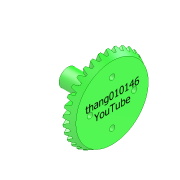
# Autodesk Inventor part: Bevel32x2i2
Saved by Autodesk Inventor 2022.5 (Build 265521000, 521)
## iProperties
Created: 2011-06-16
Part Number: Bevel32x2i2
Document SubType Name: Modeling
Designer: nguyenducthang
Density: 1 g/cm^3
Mass: 34.1157 g
Surface Area: 133.346 cm^2
Volume: 34.1157 cm^3
Material: Generic
Appearance: LED - Green On
Author: nguyenducthang
Autodesk Inventor part; units mm, degrees
ref_plane "YZ Plane" through (0, 0, 0) normal (1, 0, 0) x (0, 1, 0)
sketch "Sketch1" plane through (0, 0, 0) normal (0, 0, 1) x (1, 0, 0)
  line L0 (0, 0) -> (18.861541, 37.723166) construction
  circle A0 centre (0, 0) radius 40 construction
  line L1 (24, 32.721366) -> (16.099657, 36.671529)
  line L2 (21.641182, 47.754605) -> (4.383231, 13.238626) construction
  line L3 (12.405483, 19.444448) -> (19.776293, 34.186101) construction
  line L4 (18, 24.541025) -> (12.073062, 27.504487)
  line L5 (16.099657, 36.671529) -> (16.077282, 36.62678)
  line L6 (0, 0) -> (32.983598, 0) construction
  line L7 (40, 0) -> (43.641618, 0) construction
  line L8 (32.983598, 0) -> (54.544317, 0)
  line L9 (16.077282, 36.62678) -> (12.073062, 27.504487)
  line L10 (18, 24.541025) -> (18, 0)
  line L11 (24, 32.721366) -> (24, 0)
  line L12 (12.073062, 27.504487) -> (0, 0) construction
  line L13 (17.888512, 35.777104) -> (33.472121, 35.777104) construction
  line L14 (17.888512, 35.777104) -> (17.888512, -0.758366) construction
  line L15 (18, 0) -> (24, 0)
  dimension "d0" = 80
  dimension "d2" = 2
  dimension "d3" = 2.4
  dimension "d5" = 10
  dimension "d9" = 40
  dimension "d74" = 63.435
  dimension "d75" = 18
  dimension "d76" = 24
  dimension "d77" = 35.7771
  dimension "d78" = 17.88851
  dimension "d109" = 6.11149
  constraints: 32 end point, 7 perpendicular, 4 collinear, 4 point on line, 3 point on circle, 2 horizontal, 1 centre point, 1 coincident, 1 parallel, 1 tangent, 1 other
  measures "d0" diameter of A0
  measures "d2" distance between parallel lines of L2 L0
  measures "d3" distance between parallel lines of L3 L0
  measures "d5" distance between parallel lines of L4 L1
  measures "d9" distance from line of L1 A0.centre
  measures "d74" angle of L6 L0
  measures "d75" distance from line of L10 A0.centre
  measures "d76" distance from line of L11 A0.centre
  measures "d77" distance between parallel lines of L13 L6
  measures "d78" distance from line of L0.start L14
  measures "d109" distance between parallel lines of L11 L14
sketch "Sketch1 outline for Revolution1" plane through (0, 0, 0) normal (0, 0, 1) x (1, 0, 0)
  line L0 (16.099657, 36.671529) -> (24, 32.721366)
  line L1 (24, 32.721366) -> (24, 0)
  line L2 (24, 0) -> (18, 0)
  line L3 (18, 0) -> (18, 24.541025)
  line L4 (18, 24.541025) -> (12.073062, 27.504487)
  line L5 (12.073062, 27.504487) -> (16.077282, 36.62678)
  line L6 (16.077282, 36.62678) -> (16.099657, 36.671529)
revolve "Revolution1" add sketch "Sketch1 outline for Revolution1" angle 360 about axis through (32.983598, 0, 0) along (1, 0, 0)
ref_plane "Work Plane7" through (17.888512, 35.777104, 0) normal (0.4472128, 0.8944276, 0) x (0, 0, 1)
ref_plane "Work Plane6" through (0, 0, 0) normal (0.4472128, 0.8944276, 0) x (0, 0, 1)
sketch "Sketch11" plane through (17.888512, 35.777104, 0) normal (0.4472128, 0.8944276, 0) x (0, 0, 1)
  ellipse E0 centre (0, 14.399977) end of major axis (36.671529, 14.399977) minor radius 16.399977
  line L0 (0, 14.399977) -> (0, -5.22706) construction
  line L1 (0, -2) -> (-19.262991, -2) construction
  line L2 (4.874148, 0) -> (-7.971764, 0) construction
  line L3 (-0.882471, 2.4) -> (0, 2.4) construction
  line L4 (-1.756, -4.812675) -> (-1.756, 0) construction
  line L5 (-0.882471, 2.4) -> (-2.665926, -2.5) construction
  line L6 (0, -2.5) -> (-2.665926, -2.5) construction
  line L7 (-2.865926, -4.57661) -> (-2.865926, -2.312298) construction
  line L8 (-1.082471, 2.959829) -> (-1.082471, 2.047346) construction
  line L9 (-0.882471, 2.4) -> (-1.082471, 2.4) construction
  line L10 (-2.665926, -2.5) -> (-2.865926, -2.5) construction
  arc A0 (-2.865926, -2.5) -> (-1.082471, 2.4) centre (-18.843115, 6.089783) ccw
  arc A1 (1.082471, 2.4) -> (2.865926, -2.5) centre (18.843115, 6.089783) ccw
  line L11 (-2.865926, -2.5) -> (2.865926, -2.5)
  line L12 (1.082471, 2.4) -> (-1.082471, 2.4)
  dimension "d88" = 1.756
  dimension "d89" = 20
  dimension "d90" = 2
  dimension "d91" = 0.5
  dimension "d92" = 2.4
  dimension "d93" = 0.2
  dimension "d94" = 0.2
  constraints: 26 end point, 7 point on line, 6 perpendicular, 5 point on circle, 3 parallel, 3 symmetric about line, 2 centre point, 2 horizontal, 1 collinear, 1 vertical, 1 vertical alignment, 2 other
  measures "d88" distance between parallel lines of L0 L4
  measures "d89" angle of L5 L0
  measures "d90" distance between parallel lines of L1 L2
  measures "d91" distance between parallel lines of L6 L1
  measures "d92" distance between parallel lines of L2 L3
  measures "d93" distance from line of L7 L5.end
  measures "d94" distance from line of L8 L3.start
sketch "Sketch11 outline for Extrusion7" plane through (17.888512, 35.777104, 0) normal (0.4472128, 0.8944276, 0) x (0, 0, 1)
  arc A0 (-2.865926, -2.5) -> (-1.082471, 2.4) centre (-18.843115, 6.089783) ccw
  line L0 (-1.082471, 2.4) -> (1.082471, 2.4)
  arc A1 (1.082471, 2.4) -> (2.865926, -2.5) centre (18.843115, 6.089783) ccw
  line L1 (2.865926, -2.5) -> (-2.865926, -2.5)
extrude "Extrusion7" cut sketch "Sketch11 outline for Extrusion7" against normal blind 12 draft -2.86
ref_plane "Work Plane8" through (17.889, 0, 0) normal (1, 0, 0) x (0, 0, -1)
sketch "Sketch13" plane through (17.889, 0, 0) normal (1, 0, 0) x (0, 0, -1)
  circle A0 centre (0, 0) radius 32.721366
  circle A1 centre (0, 0) radius 35.7775
  dimension "d111" = 71.555
  constraints: 1 centre point, 1 coincident
  measures "d111" diameter of A1
sketch "Sketch14" plane through (24, 0, 0) normal (1, 0, 0) x (0, 0, -1)
  circle A0 centre (0, 0) radius 32.721366
  circle A1 centre (0, 0) radius 17 construction
  circle A2 centre (0, 17) radius 6
  dimension "d112" = 34
  dimension "d113" = 12
  constraints: 1 centre point, 1 coincident, 1 vertical alignment, 2 other
  measures "d113" diameter of A2
extrude "Extrusion9" [suppressed]
pattern_circular "Circular Pattern4" [suppressed]
pattern_circular "Circular Pattern5" count 32 over 360 about axis through (20.049828, 0, 0) along (1, 0, 0) of "Extrusion7"
sketch "Sketch15" plane through (18, 0, 0) normal (-1, 0, 0) x (0, 0, 1)
  circle A0 centre (0, 0) radius 15
  dimension "d122" = 30
  constraints: 1 centre point, 1 coincident
  measures "d122" diameter of A0
sketch "Sketch15 outline for Extrusion10" plane through (18, 0, 0) normal (-1, 0, 0) x (0, 0, 1)
  circle A0 centre (0, 0) radius 15
extrude "Extrusion10" add sketch "Sketch15 outline for Extrusion10" along normal blind 2
sketch "Sketch16" plane through (16, 0, 0) normal (-1, 0, 0) x (0, 0, 1)
  circle A0 centre (0, 0) radius 8
  dimension "d125" = 16
  constraints: 1 centre point, 1 coincident
  measures "d125" diameter of A0
sketch "Sketch16 outline for Extrusion11" plane through (16, 0, 0) normal (-1, 0, 0) x (0, 0, 1)
  circle A0 centre (0, 0) radius 8
extrude "Extrusion11" add sketch "Sketch16 outline for Extrusion11" along normal blind 32
sketch "Sketch17" plane through (24, 0, 0) normal (1, 0, 0) x (0, 0, -1)
  line L0 (-24.04849, 9.05053) -> (3.874929, 9.05053) construction
  line L1 (3.874929, 9.05053) -> (3.874929, -0.441868) construction
  line L2 (3.874929, -0.441868) -> (-24.04849, -0.441868) construction
  line L3 (-24.04849, -0.441868) -> (-24.04849, 9.05053) construction
  constraints: 2 other
sketch "Sketch18" plane through (24, 0, 0) normal (1, 0, 0) x (0, 0, -1)
  line L0 (0, 0) -> (0, 20) construction
  circle A0 centre (0, 20) radius 2.5
  dimension "d128" = 5
  dimension "d129" = 20
  constraints: 2 end point, 1 centre point, 1 coincident, 1 vertical
  measures "d128" diameter of A0
  measures "d129" distance of L0.start L0.end
sketch "Sketch18 outline for Extrusion12" plane through (24, 0, 0) normal (1, 0, 0) x (0, 0, -1)
  circle A0 centre (0, 20) radius 2.5
extrude "Extrusion12" cut sketch "Sketch18 outline for Extrusion12" against normal blind 6
pattern_circular "Circular Pattern6" count 4 over 360 about axis through (20.049828, 0, 0) along (1, 0, 0) of "Extrusion12"
body "Solid1"
